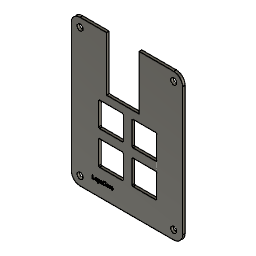
frontcase (Autodesk Fusion 360 design; units mm, degrees)
part number: 2026-02-03-18-00-08-710
Autodesk Fusion 360 part; units mm, degrees
sketch "plate-2026-02-03T10_45_19.917Z" plane through (0, 0, 0) normal (0, 1, 0) x (1, 0, 0)
  line L0 (3.025, -2.525) -> (16.025, -2.525)
  line L1 (3.025, -16.525) -> (16.025, -16.525)
  line L2 (2.525, -3.025) -> (2.525, -16.025)
  line L3 (16.525, -3.025) -> (16.525, -16.025)
  arc A0 (3.025, -2.525) -> (2.525, -3.025) centre (3.025, -3.025) ccw
  arc A1 (16.525, -3.025) -> (16.025, -2.525) centre (16.025, -3.025) ccw
  arc A2 (2.525, -16.025) -> (3.025, -16.525) centre (3.025, -16.025) ccw
  arc A3 (16.025, -16.525) -> (16.525, -16.025) centre (16.025, -16.025) ccw
  line L4 (22.075, -2.525) -> (35.075, -2.525)
  line L5 (22.075, -16.525) -> (35.075, -16.525)
  line L6 (21.575, -3.025) -> (21.575, -16.025)
  line L7 (35.575, -3.025) -> (35.575, -16.025)
  arc A4 (22.075, -2.525) -> (21.575, -3.025) centre (22.075, -3.025) ccw
  arc A5 (35.575, -3.025) -> (35.075, -2.525) centre (35.075, -3.025) ccw
  arc A6 (21.575, -16.025) -> (22.075, -16.525) centre (22.075, -16.025) ccw
  arc A7 (35.075, -16.525) -> (35.575, -16.025) centre (35.075, -16.025) ccw
  line L8 (3.025, -21.575) -> (16.025, -21.575)
  line L9 (3.025, -35.575) -> (16.025, -35.575)
  line L10 (2.525, -22.075) -> (2.525, -35.075)
  line L11 (16.525, -22.075) -> (16.525, -35.075)
  arc A8 (3.025, -21.575) -> (2.525, -22.075) centre (3.025, -22.075) ccw
  arc A9 (16.525, -22.075) -> (16.025, -21.575) centre (16.025, -22.075) ccw
  arc A10 (2.525, -35.075) -> (3.025, -35.575) centre (3.025, -35.075) ccw
  arc A11 (16.025, -35.575) -> (16.525, -35.075) centre (16.025, -35.075) ccw
  line L12 (22.075, -21.575) -> (35.075, -21.575)
  line L13 (22.075, -35.575) -> (35.075, -35.575)
  line L14 (21.575, -22.075) -> (21.575, -35.075)
  line L15 (35.575, -22.075) -> (35.575, -35.075)
  arc A12 (22.075, -21.575) -> (21.575, -22.075) centre (22.075, -22.075) ccw
  arc A13 (35.575, -22.075) -> (35.075, -21.575) centre (35.075, -22.075) ccw
  arc A14 (21.575, -35.075) -> (22.075, -35.575) centre (22.075, -35.075) ccw
  arc A15 (35.075, -35.575) -> (35.575, -35.075) centre (35.075, -35.075) ccw
sketch "Sketch2" plane through (0, 0, 0) normal (0, 1, 0) x (1, 0, 0)
  line L0 (-13.007, -70.786) -> (50.214, -70.786)
  line L1 (50.214, -70.786) -> (50.214, 12.214)
  line L2 (50.214, 12.214) -> (-13.007, 12.214)
  line L3 (-13.007, 12.214) -> (-13.007, -70.786)
  line L4 (2.525, -3.025) -> (2.525, -16.025)
  line L5 (3.025, -2.525) -> (16.025, -2.525)
  line L6 (7.03, -71) -> (25.53, -71)
  line L7 (25.53, -71) -> (25.53, -40)
  line L8 (25.53, -40) -> (7.03, -40)
  line L9 (7.03, -40) -> (7.03, -71)
  circle A0 centre (45.214, -65.786) radius 1.7
  circle A1 centre (45.214, 7.214) radius 1.7
  circle A2 centre (-8.007, 7.214) radius 1.7
  circle A3 centre (-8.007, -65.786) radius 1.7
  dimension "d1" = 83
  dimension "d2" = 63.221
  dimension "d3" = 15.532
  dimension "d4" = 14.739
  dimension "d5" = 18.5
  dimension "d6" = 31
  dimension "d7" = 20.037
  dimension "d8" = 3.4
  dimension "d9" = 5
  dimension "d10" = 5
  dimension "d11" = 3.4
  dimension "d12" = 3.4
  dimension "d13" = 3.4
  dimension "d14" = 5
  dimension "d15" = 5
  dimension "d16" = 5
  dimension "d17" = 5
  dimension "d18" = 5
  dimension "d19" = 5
  constraint horizontal L0
  constraint vertical L1
  constraint horizontal L2
  constraint vertical L3
  constraint horizontal L6
  constraint vertical L7
  constraint horizontal L8
  constraint vertical L9
  measures "d1" distance of L0.start L2.end
  measures "d2" distance of L1 L3
  measures "d3" distance of L3 L4
  measures "d4" distance of L2 L5
  measures "d5" distance of L6.start L6.end
  measures "d6" distance of L6.start L8.end
  measures "d7" distance of L3 L9
  measures "d8" diameter of A0
  measures "d9" distance of L1 A0.centre
  measures "d10" distance of L0 A0.centre
  measures "d11" diameter of A1
  measures "d12" diameter of A2
  measures "d13" diameter of A3
  measures "d14" distance of L0 A3.centre
  measures "d15" distance of L3 A3.centre
  measures "d16" distance of L3 A2.centre
  measures "d17" distance of L2 A2.centre
  measures "d18" distance of L2 A1.centre
  measures "d19" distance of L1 A1.centre
sketch "Sketch3" plane through (0, 0, 0) normal (0, 1, 0) x (1, 0, 0)
extrude "Extrude1" add sketch "Sketch2" along normal blind 1.5 contours L0 L1 L2 L3 L7 L8 L9
extrude "Extrude2" cut sketch "plate-2026-02-03T10_45_19.917Z" along normal blind 1.5
fillet "Fillet1" radius 5 1 edges at (50.214, 0.75, 70.786)
fillet "Fillet2" radius 5 1 edges at (-13.007, 0.75, 70.786)
fillet "Fillet3" radius 5 1 edges at (-13.007, 0.75, -12.214)
fillet "Fillet4" radius 5 1 edges at (50.214, 0.75, -12.214)
sketch "Sketch4" plane through (0, 0, 0) normal (0, 1, 0) x (1, 0, 0)
  line L0 (-0.9253, 10.0676) -> (13.6705, 10.1334) construction
  line L1 (13.6705, 10.1334) -> (13.7027, 2.985) construction
  line L2 (13.7027, 2.985) -> (-0.893, 2.9193) construction
  line L3 (-0.893, 2.9193) -> (-0.9253, 10.0676) construction
  dimension "d32" = 2
  text T0 "LayaCore" font "Arial" height 2 align left top in box 14.5959 x 7.1484 at (-0.9253, 10.0676) x (0.99999, 0.004506) y (0.004506, -0.99999) spacing 1
extrude "Extrude3" add sketch "Sketch4" against normal blind 0.2 text T0
equation "d33 = 'LayaCore'"
